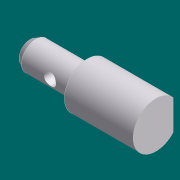
# Autodesk Inventor part: P12
Saved by Autodesk Inventor 2012 SP1 (Build 160190100, 190)
## iProperties
Created: 2011-06-16
Part Number: P12
Material: Aluminium
Document SubType Name: Modeling
Designer: sta
Density: 2.7 g/cm^3
Description: Welle
Mass: 1.9886 g
Surface Area: 5.61547 cm^2
Volume: 0.736518 cm^3
Title: Kart
Author: sta
Autodesk Inventor part; units mm, degrees
ref_plane "YZ Plane" through (0, 0, 0) normal (1, 0, 0) x (0, 1, 0)
ref_plane "XY Plane" through (0, 0, 0) normal (0, 0, 1) x (1, 0, 0)
sketch "Sketch1" plane through (0, 0, 0) normal (0, 0, 1) x (1, 0, 0)
  line L0 (0, 0) -> (51.053, 0) construction
  line L1 (0, 0) -> (0, 2.5)
  line L2 (0, 2.5) -> (10, 2.5)
  line L3 (10, 2.5) -> (10, 4)
  line L4 (10, 4) -> (22, 4)
  line L5 (22, 4) -> (22, 0)
  line L6 (22, 0) -> (0, 0)
  dimension "d0" = 5
  dimension "d1" = 8
  dimension "d2" = 10
  dimension "d3" = 12
  constraints: 14 end point, 3 perpendicular, 2 parallel, 1 coincident, 1 collinear, 1 horizontal, 1 point on line
  measures "d0" diameter of L2 L0
  measures "d1" diameter of L4 L0
  measures "d2" distance from line of L3 L1.end
  measures "d3" distance between parallel lines of L5 L3
revolve "Revolution1" add sketch "Sketch1" angle 360 about axis through (0, 0, 0) along (1, 0, 0)
sketch "Sketch2" plane through (22, 0, 0) normal (1, 0, 0) x (0, 0, -1)
  circle A0 centre (0, 0) radius 4 projected
  circle A1 centre (0, 0) radius 2.5 construction
  line L0 (-2.6458, 3) -> (2.6458, 3)
  arc A2 (2.6458, 3) -> (-2.6458, 3) centre (0, 0) ccw
  dimension "d5" = 3
  constraints: 4 point on circle, 2 end point, 1 centre point, 1 coincident, 1 horizontal
  measures "d5" distance from line of L0 point (0, 0)
extrude "Extrusion1" cut sketch "Sketch2" against normal through all contours L0 A0 picked at (-0.6179, 3.1815)
ref_plane "Work Plane1" through (5, 2.5, 0) normal (0, 1, 0) x (-1, 0, 0)
sketch "Sketch3" plane through (5, 2.5, 0) normal (0, 1, 0) x (-1, 0, 0)
  line L0 (-5, 2.5) -> (-5, -2.5) construction
  line L1 (5, 2.5) -> (5, -2.5) construction
  line L2 (-5, 2.6458) -> (-5, -2.6458) construction
  line L3 (-5, 0) -> (5, 0) construction
  point P0 (-1, 0)
  dimension "d8" = 4
  constraints: 2 end point, 1 midpoint, 1 perpendicular, 1 point on line
  measures "d8" distance from line of point (-1, 0) L0
hole "Hole1" at (6, 2.5, 0) direction (0, -1, 0) diameter 2 end through all
chamfer "Chamfer1" distance 1 angle 30 1 edges at (0, -2.5, 0) measured on face at (5.3098, -2.0345, -1.4529)
body "Solid1"
